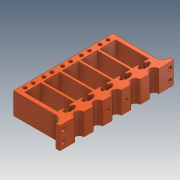
# Autodesk Inventor part: servo-holder-1
Saved by Autodesk Inventor 2017 (Build 210142000, 142)
## iProperties
Created: 2018-05-30
Part Number: servo-holder-1
Material: Generic
Document SubType Name: Modeling
Designer: Luiz Gustavo
Density: 1 g/cm^3
Appearance: Smooth - Light Orange
Author: Luiz Gustavo
Autodesk Inventor part; units mm, degrees
ref_plane "YZ Plane" through (0, 0, 0) normal (1, 0, 0) x (0, 1, 0)
ref_plane "XZ Plane" through (0, 0, 0) normal (0, 1, 0) x (-1, 0, 0)
ref_plane "XY Plane" through (0, 0, 0) normal (0, 0, 1) x (1, 0, 0)
sketch "Sketch1" plane through (0, 0, 0) normal (0, 0, 1) x (1, 0, 0)
  line L0 (-20.4, -10.1) -> (20.4, -10.1)
  line L1 (20.4, -10.1) -> (20.4, 10.1)
  line L2 (20.4, 10.1) -> (-20.4, 10.1)
  line L3 (-20.4, 10.1) -> (-20.4, -10.1)
  line L4 (-20.4, -10.1) -> (20.4, 10.1) construction
  line L5 (20.4, -10.1) -> (-20.4, 10.1) construction
  line L6 (-20.4, 13.1) -> (20.4, 13.1)
  line L7 (20.4, 13.1) -> (20.4, 33.3)
  line L8 (20.4, 33.3) -> (-20.4, 33.3)
  line L9 (-20.4, 33.3) -> (-20.4, 13.1)
  line L10 (-20.4, 13.1) -> (20.4, 33.3) construction
  line L11 (20.4, 13.1) -> (-20.4, 33.3) construction
  line L12 (-20.4, 36.3) -> (20.4, 36.3)
  line L13 (20.4, 36.3) -> (20.4, 56.5)
  line L14 (20.4, 56.5) -> (-20.4, 56.5)
  line L15 (-20.4, 56.5) -> (-20.4, 36.3)
  line L16 (-20.4, 36.3) -> (20.4, 56.5) construction
  line L17 (20.4, 36.3) -> (-20.4, 56.5) construction
  line L18 (-20.4, -13.1) -> (20.4, -13.1)
  line L19 (20.4, -13.1) -> (20.4, -33.3)
  line L20 (20.4, -33.3) -> (-20.4, -33.3)
  line L21 (-20.4, -33.3) -> (-20.4, -13.1)
  line L22 (-20.4, -13.1) -> (20.4, -33.3) construction
  line L23 (20.4, -13.1) -> (-20.4, -33.3) construction
  line L24 (-20.4, -36.3) -> (20.4, -36.3)
  line L25 (20.4, -36.3) -> (20.4, -56.5)
  line L26 (20.4, -56.5) -> (-20.4, -56.5)
  line L27 (-20.4, -56.5) -> (-20.4, -36.3)
  line L28 (-20.4, -36.3) -> (20.4, -56.5) construction
  line L29 (20.4, -36.3) -> (-20.4, -56.5) construction
  line L30 (0, 46.4) -> (0, -46.4) construction
  line L31 (20.4, -10.1) -> (20.4, -13.1) construction
  line L32 (20.4, 0) -> (20.4, 10.1) construction
  line L33 (20.4, -33.3) -> (20.4, -36.3) construction
  line L34 (20.4, -13.1) -> (20.4, -33.3) construction
  line L35 (20.4, 33.3) -> (20.4, 36.3) construction
  line L36 (20.4, 36.3) -> (20.4, 56.5) construction
  line L37 (20.4, 10.1) -> (20.4, 13.1) construction
  line L38 (-29, 61.5) -> (29, 61.5)
  line L39 (29, 61.5) -> (29, -61.5)
  line L40 (29, -61.5) -> (-29, -61.5)
  line L41 (-29, -61.5) -> (-29, 61.5)
  line L42 (-29, 61.5) -> (29, -61.5) construction
  line L43 (29, 61.5) -> (-29, -61.5) construction
  line L44 (29, -61.5) -> (37.3, -61.5)
  line L45 (37.3, -61.5) -> (37.3, -52.15)
  line L46 (37.3, 61.5) -> (29, 61.5)
  line L47 (29, 61.5) -> (29, -61.5)
  arc A0 (37.3, -40.65) -> (37.3, -52.15) centre (37.3, -46.4) ccw
  line L48 (0, -46.4) -> (37.3, -46.4) construction
  arc A1 (37.3, -17.45) -> (37.3, -28.95) centre (37.3, -23.2) ccw
  arc A2 (37.3, 5.75) -> (37.3, -5.75) centre (37.3, 0) ccw
  arc A3 (37.3, 28.95) -> (37.3, 17.45) centre (37.3, 23.2) ccw
  arc A4 (37.3, 52.15) -> (37.3, 40.65) centre (37.3, 46.4) ccw
  line L49 (0, -23.2) -> (37.3, -23.2) construction
  line L50 (0, 46.4) -> (37.3, 46.4) construction
  line L51 (0, 23.2) -> (37.3, 23.2) construction
  line L52 (0, 0) -> (37.3, 0) construction
  arc A5 (37.3, -52.15) -> (37.3, -40.65) centre (37.3, -46.4) ccw construction
  arc A6 (37.3, -28.95) -> (37.3, -17.45) centre (37.3, -23.2) ccw construction
  arc A7 (37.3, -5.75) -> (37.3, 5.75) centre (37.3, 0) ccw construction
  arc A8 (37.3, 17.45) -> (37.3, 28.95) centre (37.3, 23.2) ccw construction
  arc A9 (37.3, 40.65) -> (37.3, 52.15) centre (37.3, 46.4) ccw construction
  line L53 (37.3, -40.65) -> (37.3, -28.95)
  line L54 (37.3, -52.15) -> (37.3, -40.65) construction
  line L55 (37.3, -28.95) -> (37.3, -17.45) construction
  line L56 (37.3, -17.45) -> (37.3, -5.75)
  line L57 (37.3, -5.75) -> (37.3, 5.75) construction
  line L58 (37.3, 5.75) -> (37.3, 17.45)
  line L59 (37.3, 28.95) -> (37.3, 40.65)
  line L60 (37.3, 17.45) -> (37.3, 28.95) construction
  line L61 (37.3, 52.15) -> (37.3, 61.5)
  line L62 (37.3, 40.65) -> (37.3, 52.15) construction
  point P0 (0, 0)
  point P1 (0, 23.2)
  point P2 (0, -23.2)
  dimension "d0" = 20.2
  dimension "d1" = 40.8
  dimension "d2" = 3
  dimension "d4" = 58
  dimension "d10" = 11.5
  dimension "d11" = 8.3
  dimension "d14" = 16.9
  dimension "d55" = 123
  constraints: 116 end point, 22 midpoint, 20 point on circle, 19 parallel, 17 horizontal, 13 vertical, 12 perpendicular, 11 collinear, 10 centre point, 8 point on line, 4 equal radius, 64 other
  measures "d0" distance of L0.end L1.end
  measures "d1" distance between parallel lines of L3 L1
  measures "d2" distance of L0.end L18.end
  measures "d4" distance of L38.start L38.end
  measures "d10" diameter of A0
  measures "d14" distance from line of L48.end L25
  measures "d55" distance between parallel lines of L38 L40
extrude "Extrusion1" add sketch "Sketch1" along normal blind 27 contours L38 L39 L40 L41
extrude "Extrusion3" add sketch "Sketch1" along normal up to surface (27 mm away) contours L46 L61 A4 L59 A3 L58 A2 L56 A1 L53 A0 L45 L44 L39
sketch "Sketch3" plane through (0, 0, 0) normal (0, 0, 1) x (1, 0, 0)
  line L0 (20.4, 56.5) -> (20.4, 36.3) projected
  line L1 (20.4, 33.3) -> (20.4, 13.1) projected
  line L2 (20.4, 10.1) -> (20.4, -10.1) projected
  line L3 (20.4, -13.1) -> (20.4, -33.3) projected
  line L4 (20.4, -36.3) -> (20.4, -56.5) projected
  circle A0 centre (25.05, 51.4) radius 2.15
  circle A1 centre (25.05, 41.4) radius 2.15
  circle A2 centre (25.05, 28.2) radius 2.15
  circle A3 centre (25.05, 18.2) radius 2.15
  circle A4 centre (25.05, 5) radius 2.15
  circle A5 centre (25.05, -5) radius 2.15
  circle A6 centre (25.05, -18.2) radius 2.15
  circle A7 centre (25.05, -28.2) radius 2.15
  circle A8 centre (25.05, -41.4) radius 2.15
  circle A9 centre (25.05, -51.4) radius 2.15
  line L5 (25.05, 51.4) -> (25.05, -51.4) construction
  line L6 (20.4, 46.4) -> (25.05, 46.4) construction
  line L7 (20.4, 23.2) -> (25.05, 23.2) construction
  line L8 (20.4, 0) -> (25.05, 0) construction
  line L9 (20.4, -23.2) -> (25.05, -23.2) construction
  line L10 (20.4, -46.4) -> (25.05, -46.4) construction
  line L11 (0.05, 51.4) -> (0.05, -53.9) construction
  circle A10 centre (-24.95, 51.4) radius 2.15
  circle A11 centre (-24.95, 41.4) radius 2.15
  circle A12 centre (-24.95, 28.2) radius 2.15
  circle A13 centre (-24.95, 18.2) radius 2.15
  circle A14 centre (-24.95, 5) radius 2.15
  circle A15 centre (-24.95, -5) radius 2.15
  circle A16 centre (-24.95, -18.2) radius 2.15
  circle A17 centre (-24.95, -28.2) radius 2.15
  circle A18 centre (-24.95, -41.4) radius 2.15
  circle A19 centre (-24.95, -51.4) radius 2.15
  point P0 (0, 0)
  dimension "d15" = 4.3
  dimension "d19" = 10
  dimension "d20" = 10
  dimension "d21" = 10
  dimension "d22" = 10
  dimension "d23" = 10
  dimension "d27" = 4.65
  dimension "d28" = 50
  constraints: 20 centre point, 12 end point, 10 symmetric about line, 9 equal radius, 5 horizontal, 5 midpoint, 2 coincident, 1 vertical, 31 other
  measures "d15" diameter of A0
  measures "d19" distance of A1.centre A0.centre
  measures "d20" distance of A3.centre A2.centre
  measures "d21" distance of A5.centre A4.centre
  measures "d22" distance of A7.centre A6.centre
  measures "d23" distance of A9.centre A8.centre
extrude "Extrusion4" cut sketch "Sketch3" along normal through all
sketch "Sketch4" plane through (0, 0, 0) normal (0, 0, 1) x (1, 0, 0)
  line L0 (20.4, -56.5) -> (20.4, -36.3) construction
  line L1 (20.4, -33.3) -> (20.4, -13.1) construction
  line L2 (20.4, -10.1) -> (20.4, 10.1) construction
  line L3 (20.4, 13.1) -> (20.4, 33.3) construction
  line L4 (20.4, 36.3) -> (20.4, 56.5) construction
  line L5 (20.4, -36.3) -> (20.4, -56.5) projected
  line L6 (20.4, -49.9) -> (28.4, -49.9)
  line L7 (28.4, -49.9) -> (28.4, -42.9)
  line L8 (28.4, -42.9) -> (20.4, -42.9)
  line L9 (20.4, -42.9) -> (20.4, -49.9)
  line L10 (28.4, -46.4) -> (20.4, -46.4) construction
  line L11 (20.4, -26.7) -> (28.4, -26.7)
  line L12 (28.4, -26.7) -> (28.4, -19.7)
  line L13 (28.4, -19.7) -> (20.4, -19.7)
  line L14 (20.4, -19.7) -> (20.4, -26.7)
  line L15 (28.4, -23.2) -> (20.4, -23.2) construction
  line L16 (20.4, -3.5) -> (28.4, -3.5)
  line L17 (28.4, -3.5) -> (28.4, 3.5)
  line L18 (28.4, 3.5) -> (20.4, 3.5)
  line L19 (20.4, 3.5) -> (20.4, -3.5)
  line L20 (28.4, 0) -> (20.4, 0) construction
  line L21 (20.4, 19.7) -> (28.4, 19.7)
  line L22 (28.4, 19.7) -> (28.4, 26.7)
  line L23 (28.4, 26.7) -> (20.4, 26.7)
  line L24 (20.4, 26.7) -> (20.4, 19.7)
  line L25 (28.4, 23.2) -> (20.4, 23.2) construction
  line L26 (20.4, 42.9) -> (28.4, 42.9)
  line L27 (28.4, 42.9) -> (28.4, 49.9)
  line L28 (28.4, 49.9) -> (20.4, 49.9)
  line L29 (20.4, 49.9) -> (20.4, 42.9)
  line L30 (28.4, 46.4) -> (20.4, 46.4) construction
  point P0 (0, 0)
  dimension "d31" = 8
  dimension "d32" = 7
  constraints: 50 end point, 15 midpoint, 10 parallel, 8 equal length, 5 horizontal, 5 perpendicular, 2 point on line
  measures "d31" distance between parallel lines of L0 L7
  measures "d32" distance between parallel lines of L8 L6
extrude "Extrusion5" cut sketch "Sketch4" along normal through all
sketch "Sketch5" plane through (0, 0, 0) normal (0, 0, 1) x (1, 0, 0)
  line L0 (-29, 61.5) -> (37.3, 61.5) projected
  line L1 (-29, -61.5) -> (37.3, -61.5) projected
  line L2 (37.3, 61.5) -> (37.3, 70.5)
  line L3 (37.3, 70.5) -> (32.3, 70.5)
  arc A0 (23.3, 61.5) -> (32.3, 70.5) centre (23.3, 70.5) ccw
  line L4 (32.3, 70.5) -> (32.3, 61.5) construction
  line L5 (-33.15, 0) -> (33.15, 0) construction
  line L6 (37.3, -61.5) -> (37.3, -70.5)
  line L7 (37.3, -70.5) -> (32.3, -70.5)
  arc A1 (32.3, -70.5) -> (23.3, -61.5) centre (23.3, -70.5) ccw
  line L8 (32.3, -70.5) -> (32.3, -61.5) construction
  line L9 (23.3, 61.5) -> (37.3, 61.5)
  line L10 (23.3, -61.5) -> (37.3, -61.5)
  point P0 (0, 0)
  point P1 (0, 0)
  dimension "d38" = 9
  dimension "d39" = 5
  constraints: 18 end point, 5 symmetric about line, 4 point on circle, 2 centre point, 2 horizontal, 2 point on line, 2 tangent, 1 coincident, 1 collinear, 1 midpoint, 1 perpendicular, 1 vertical, 1 other
  measures "d38" distance of L0.end L2.end
  measures "d39" distance of L2.end L3.end
extrude "Extrusion6" add sketch "Sketch5" along normal up to surface (27 mm away)
sketch "Sketch6" plane through (0, 0, 0) normal (1, 0, 0) x (0, 1, 0)
  line L0 (-52.15, 27) -> (-70.5, 27) projected
  line L1 (-70.5, 0) -> (-70.5, 27) projected
  line L2 (-61.5, 0) -> (-61.5, 27) projected
  circle A0 centre (-66, 20.1625) radius 4.5
  circle A1 centre (-66, 20.1625) radius 2.6
  line L3 (-70.5, 13.5) -> (-61.5, 13.5) construction
  circle A2 centre (-66, 6.8375) radius 4.5
  circle A3 centre (-66, 6.8375) radius 2.6
  line L4 (0, 0) -> (0, 27) construction
  circle A4 centre (66, 20.1625) radius 4.5
  circle A5 centre (66, 20.1625) radius 2.6
  circle A6 centre (66, 6.8375) radius 4.5
  circle A7 centre (66, 6.8375) radius 2.6
  dimension "d43" = 5.2
  dimension "d46" = 2.3375
  dimension "d47" = 4.325
  dimension "d59" = 9
  constraints: 8 centre point, 6 symmetric about line, 4 coincident, 4 end point, 2 midpoint, 1 tangent, 1 vertical, 6 other
  measures "d43" diameter of A1
  measures "d46" distance edge to line of A0 L0
  measures "d59" diameter of A0
extrude "Extrusion7" cut sketch "Sketch6" along normal through all contours A1 | A3 | A5 | A7
extrude "Extrusion8" cut sketch "Sketch6" along normal blind 32 contours A0 | A2 | A4 | A6
chamfer "Chamfer1" [suppressed]
sketch "Sketch7" plane through (37.3, 5.75, 0) normal (1, 0, 0) x (0, 0, -1)
  line L0 (-27, -11.5) -> (-27, -23.2) projected
  line L1 (0, -23.2) -> (-27, -23.2) projected
  line L2 (0, -23.2) -> (0, -11.5) projected
  line L3 (0, -11.5) -> (-27, -11.5) projected
  line L4 (-27, 11.7) -> (-27, 0) projected
  line L5 (0, 0) -> (-27, 0) projected
  line L6 (0, 0) -> (0, 11.7) projected
  line L7 (0, 11.7) -> (-27, 11.7) projected
  line L8 (0, -23.2) -> (-27, -23.2) construction
  line L9 (-13.5, -23.2) -> (-13.5, -11.5) construction
  line L10 (0, 0) -> (-27, 0) construction
  line L11 (-13.5, 0) -> (-13.5, 11.7) construction
  circle A0 centre (-13.5, 5.85) radius 2.15
  circle A1 centre (-13.5, -17.35) radius 2.15
  point P0 (0, -5.75)
  dimension "d56" = 4.3
  constraints: 6 midpoint, 4 end point, 2 centre point, 1 equal radius
  measures "d56" diameter of A0
extrude "Extrusion9" cut sketch "Sketch7" against normal blind 12 contours A0 | A1
equation "\"d20\" = d19"
equation "\"d21\" = d19"
equation "\"d22\" = d19"
equation "\"d23\" = d19"
body "Solid1"
